Autodesk Fusion 360 part; units mm, degrees
(part 2 of 3)
sketch "Road Junction Left" plane through (0, 0, 0) normal (0, 0, 1) x (1, 0, 0) in component "Road Juntcion left"
  line L0 (106.7005, 11.7668) -> (99.7723, -0.2332)
  line L1 (120.6146, 11.8668) -> (106.6427, 11.8668)
  line L2 (106.7005, -12.2332) -> (120.5569, -12.2332)
  line L3 (104.1544, -16.6432) -> (123.103, -16.6432)
  line L4 (120.0373, -11.3332) -> (126.4458, -0.2332)
  line L5 (99.6568, -0.2332) -> (106.6427, -12.3332)
  line L6 (94.68, -0.2332) -> (104.1544, -16.6432)
  line L7 (100.8115, -0.2332) -> (107.2201, -11.3332)
  line L8 (107.2201, -11.3332) -> (120.0373, -11.3332)
  line L9 (132.5773, -0.2332) -> (123.103, 16.1768)
  line L10 (127.4851, -0.2332) -> (120.5569, 11.7668)
  line L11 (124.021, 5.7668) -> (103.2364, -6.2332) construction
  line L12 (104.1544, 16.1768) -> (94.68, -0.2332)
  line L13 (103.1498, 5.8168) -> (124.1076, -6.2832) construction
  line L14 (106.6427, -12.3332) -> (120.6146, -12.3332)
  line L15 (120.6146, -12.3332) -> (127.6005, -0.2332)
  line L16 (120.5569, 11.7668) -> (106.7005, 11.7668)
  line L17 (127.6005, -0.2332) -> (120.6146, 11.8668)
  line L18 (123.103, -16.6432) -> (132.5773, -0.2332)
  line L19 (123.103, 16.1768) -> (104.1544, 16.1768)
  line L20 (126.4458, -0.2332) -> (120.0373, 10.8668)
  line L21 (120.5569, -12.2332) -> (127.4851, -0.2332)
  line L22 (106.6427, 11.8668) -> (99.6568, -0.2332)
  line L23 (120.0373, 10.8668) -> (107.2201, 10.8668)
  line L24 (113.6287, 11.7668) -> (113.6287, -12.2332) construction
  line L25 (107.2201, 10.8668) -> (100.8115, -0.2332)
  line L26 (99.7723, -0.2332) -> (106.7005, -12.2332)
  line L27 (101.5158, -1.453) -> (120.7416, 9.647)
  line L28 (106.5158, -10.1133) -> (125.7416, 0.9867)
  line L29 (101.7158, -1.7994) -> (120.9416, 9.3006)
  line L30 (106.3158, -9.7669) -> (125.5416, 1.3331)
  line L31 (118.6287, 10.8668) -> (118.6287, -11.3332)
  line L32 (108.6287, 10.8668) -> (108.6287, -11.3332)
  line L33 (118.2287, 10.8668) -> (118.2287, -11.3332)
  line L34 (109.0287, 10.8668) -> (109.0287, -11.3332)
  point P0 (113.6287, -0.2332)
  dimension "d328_3_1" = 0.1
  dimension "d330_3_1" = 32.82
  dimension "d366_1_1" = 10
  dimension "d369_1_1" = 0.4
  dimension "d421" = 10
  dimension "d422" = 0.4
  constraint horizontal L19
  constraint midpoint L24.start L16
  constraint midpoint L24.end L2
  constraint midpoint L11.start L10
  constraint midpoint L11.end L26
  constraint midpoint L13.start L22
  constraint midpoint L13.end L15
  constraint coincident L7 L27.start
  constraint coincident L20 L27.end
  constraint perpendicular L20 L27
  constraint coincident L7 L28.start
  constraint coincident L20 L28.end
  constraint perpendicular L20 L28
  constraint symmetric L11 L27 L28
  constraint coincident L23 L31.start
  constraint coincident L8 L31.end
  constraint perpendicular L8 L31
  constraint coincident L23 L32.start
  constraint coincident L8 L32.end
  constraint perpendicular L8 L32
  constraint symmetric L24 L31 L32
  measures "d330_3_1" distance of L3 L19
  measures "d366_1_1" distance of L27 L28
  measures "d421" distance of L31 L32
extrude "Cap body'" add sketch "Road Junction Left" along normal blind 4.8 separate body contours L0 L2 L10 L16 L21 L26 | L1 L5 L14 L15 L17 L22 | L3 L6 L9 L12 L18 L19 | L4 L8 L20 L28 L31 | L8 L28 L31 L33 | L20 L28 L30 L31 | L8 L28 L33 L34 | L28 L30 L31 L33 | L20 L29 L30 L31 | L8 L28 L32 L34 | L28 L30 L33 L34 | L29 L30 L31 L33 | L20 L27 L29 L31 | L7 L8 L28 L32 | L28 L30 L32 L34 | L29 L30 L33 L34 | L27 L29 L31 L33 | L20 L23 L27 L31 | L7 L28 L30 L32 | L29 L30 L32 L34 | L27 L29 L33 L34 | L23 L27 L31 L33 | L7 L29 L30 L32 | L27 L29 L32 L34 | L23 L27 L33 L34 | L7 L27 L29 L32 | L23 L27 L32 L34 | L7 L23 L25 L27 L32 makes body 9 in component "Road Juntcion left"
extrude "top lip cut''''" cut sketch "Road Junction Left" against normal blind 1.8 from surface at 4.8 contours L1 L5 L14 L15 L17 L22 | L3 L6 L9 L12 L18 L19 bodies 9 in component "Road Juntcion left"
extrude "Cap internal hole'" cut sketch "Road Junction Left" along normal blind 2 contours L0 L2 L10 L16 L21 L26 | L1 L5 L14 L15 L17 L22 | L4 L8 L20 L28 L31 | L8 L28 L31 L33 | L20 L28 L30 L31 | L8 L28 L33 L34 | L28 L30 L31 L33 | L20 L29 L30 L31 | L8 L28 L32 L34 | L28 L30 L33 L34 | L29 L30 L31 L33 | L20 L27 L29 L31 | L7 L8 L28 L32 | L28 L30 L32 L34 | L29 L30 L33 L34 | L27 L29 L31 L33 | L20 L23 L27 L31 | L7 L28 L30 L32 | L29 L30 L32 L34 | L27 L29 L33 L34 | L23 L27 L31 L33 | L7 L29 L30 L32 | L27 L29 L32 L34 | L23 L27 L33 L34 | L7 L27 L29 L32 | L23 L27 L32 L34 | L7 L23 L25 L27 L32 bodies 9 in component "Road Juntcion left"
extrude "road cut'''" cut sketch "Road Junction Left" against normal blind 1.2 from surface at 4.8 contours L4 L8 L20 L28 L31 | L8 L28 L31 L33 | L8 L28 L33 L34 | L8 L28 L32 L34 | L7 L8 L28 L32 | L20 L23 L27 L31 | L7 L23 L25 L27 L32 bodies 9 in component "Road Juntcion left"
extrude "Road depth cut" cut sketch "Road Junction Left" against normal blind 0.4 from surface at 4.8 contours L20 L29 L30 L31 | L29 L30 L31 L33 | L29 L30 L33 L34 | L29 L30 L32 L34 | L27 L29 L33 L34 | L7 L29 L30 L32 | L23 L27 L33 L34 bodies 9 in component "Road Juntcion left"
sketch "Road Junction X" plane through (0, 0, 0) normal (0, 0, 1) x (1, 0, 0) in component "Road Juntcion X"
  line L0 (106.7005, 11.7668) -> (99.7723, -0.2332)
  line L1 (120.6146, 11.8668) -> (106.6427, 11.8668)
  line L2 (106.7005, -12.2332) -> (120.5569, -12.2332)
  line L3 (104.1544, -16.6432) -> (123.103, -16.6432)
  line L4 (120.0373, -11.3332) -> (126.4458, -0.2332)
  line L5 (99.6568, -0.2332) -> (106.6427, -12.3332)
  line L6 (94.68, -0.2332) -> (104.1544, -16.6432)
  line L7 (100.8115, -0.2332) -> (107.2201, -11.3332)
  line L8 (107.2201, -11.3332) -> (120.0373, -11.3332)
  line L9 (132.5773, -0.2332) -> (123.103, 16.1768)
  line L10 (127.4851, -0.2332) -> (120.5569, 11.7668)
  line L11 (124.021, 5.7668) -> (103.2364, -6.2332) construction
  line L12 (104.1544, 16.1768) -> (94.68, -0.2332)
  line L13 (103.1498, 5.8168) -> (124.1076, -6.2832) construction
  line L14 (106.6427, -12.3332) -> (120.6146, -12.3332)
  line L15 (120.6146, -12.3332) -> (127.6005, -0.2332)
  line L16 (120.5569, 11.7668) -> (106.7005, 11.7668)
  line L17 (127.6005, -0.2332) -> (120.6146, 11.8668)
  line L18 (123.103, -16.6432) -> (132.5773, -0.2332)
  line L19 (123.103, 16.1768) -> (104.1544, 16.1768)
  line L20 (126.4458, -0.2332) -> (120.0373, 10.8668)
  line L21 (120.5569, -12.2332) -> (127.4851, -0.2332)
  line L22 (106.6427, 11.8668) -> (99.6568, -0.2332)
  line L23 (120.0373, 10.8668) -> (107.2201, 10.8668)
  line L24 (113.6287, 11.7668) -> (113.6287, -12.2332) construction
  line L25 (107.2201, 10.8668) -> (100.8115, -0.2332)
  line L26 (99.7723, -0.2332) -> (106.7005, -12.2332)
  line L27 (101.5158, -1.453) -> (120.7416, 9.647)
  line L28 (106.5158, -10.1133) -> (125.7416, 0.9867)
  line L29 (101.7158, -1.7994) -> (120.9416, 9.3006)
  line L30 (106.3158, -9.7669) -> (125.5416, 1.3331)
  line L31 (118.6287, 10.8668) -> (118.6287, -11.3332)
  line L32 (108.6287, 10.8668) -> (108.6287, -11.3332)
  line L33 (118.2287, 10.8668) -> (118.2287, -11.3332)
  line L34 (109.0287, 10.8668) -> (109.0287, -11.3332)
  point P0 (113.6287, -0.2332)
  dimension "d328_3_1_1" = 0.1
  dimension "d330_3_1_1" = 32.82
  dimension "d366_1_1_1" = 10
  dimension "d369_1_1_1" = 0.4
  dimension "d421_1" = 10
  dimension "d422_1" = 0.4
  constraint horizontal L19
  constraint midpoint L24.start L16
  constraint midpoint L24.end L2
  constraint midpoint L11.start L10
  constraint midpoint L11.end L26
  constraint midpoint L13.start L22
  constraint midpoint L13.end L15
  constraint coincident L7 L27.start
  constraint coincident L20 L27.end
  constraint perpendicular L20 L27
  constraint coincident L7 L28.start
  constraint coincident L20 L28.end
  constraint perpendicular L20 L28
  constraint symmetric L11 L27 L28
  constraint coincident L23 L31.start
  constraint coincident L8 L31.end
  constraint perpendicular L8 L31
  constraint coincident L23 L32.start
  constraint coincident L8 L32.end
  constraint perpendicular L8 L32
  constraint symmetric L24 L31 L32
  measures "d330_3_1_1" distance of L3 L19
  measures "d366_1_1_1" distance of L27 L28
  measures "d421_1" distance of L31 L32
extrude "Cap body''" add sketch "Road Junction X" along normal blind 4.8 separate body contours L0 L2 L10 L16 L21 L26 | L1 L5 L14 L15 L17 L22 | L3 L6 L9 L12 L18 L19 | L4 L8 L20 L28 L31 | L8 L28 L31 L33 | L20 L28 L30 L31 | L8 L28 L33 L34 | L28 L30 L31 L33 | L20 L29 L30 L31 | L8 L28 L32 L34 | L28 L30 L33 L34 | L29 L30 L31 L33 | L20 L27 L29 L31 | L7 L8 L28 L32 | L28 L30 L32 L34 | L29 L30 L33 L34 | L27 L29 L31 L33 | L20 L23 L27 L31 | L7 L28 L30 L32 | L29 L30 L32 L34 | L27 L29 L33 L34 | L23 L27 L31 L33 | L7 L29 L30 L32 | L27 L29 L32 L34 | L23 L27 L33 L34 | L7 L27 L29 L32 | L23 L27 L32 L34 | L7 L23 L25 L27 L32 makes body 10 in component "Road Juntcion X"
extrude "top lip cut'''''" cut sketch "Road Junction X" against normal blind 1.8 from surface at 4.8 contours L1 L5 L14 L15 L17 L22 | L3 L6 L9 L12 L18 L19 bodies 10 in component "Road Juntcion X"
extrude "Cap internal hole''" cut sketch "Road Junction X" along normal blind 2 contours L0 L2 L10 L16 L21 L26 | L1 L5 L14 L15 L17 L22 | L4 L8 L20 L28 L31 | L8 L28 L31 L33 | L20 L28 L30 L31 | L8 L28 L33 L34 | L28 L30 L31 L33 | L20 L29 L30 L31 | L8 L28 L32 L34 | L28 L30 L33 L34 | L29 L30 L31 L33 | L20 L27 L29 L31 | L7 L8 L28 L32 | L28 L30 L32 L34 | L29 L30 L33 L34 | L27 L29 L31 L33 | L20 L23 L27 L31 | L7 L28 L30 L32 | L29 L30 L32 L34 | L27 L29 L33 L34 | L23 L27 L31 L33 | L7 L29 L30 L32 | L27 L29 L32 L34 | L23 L27 L33 L34 | L7 L27 L29 L32 | L23 L27 L32 L34 | L7 L23 L25 L27 L32 bodies 10 in component "Road Juntcion X"
extrude "road cut''''" cut sketch "Road Junction X" against normal blind 1.2 from surface at 4.8 contours L4 L8 L20 L28 L31 | L7 L8 L28 L32 | L20 L23 L27 L31 | L7 L23 L25 L27 L32 bodies 10 in component "Road Juntcion X"
extrude "Extrude17" cut sketch "Road Junction X" against normal blind 0.4 from surface at 4.8 contours L8 L28 L33 L34 | L20 L29 L30 L31 | L28 L30 L33 L34 | L29 L30 L31 L33 | L29 L30 L33 L34 | L29 L30 L32 L34 | L27 L29 L33 L34 | L7 L29 L30 L32 | L23 L27 L33 L34 bodies 10 in component "Road Juntcion X"
sketch "Road Junction Y" plane through (0, 0, 0) normal (0, 0, 1) x (1, 0, 0) in component "Road Juntcion Y"
  line L0 (106.6902, 11.7491) -> (99.762, -0.2509)
  line L1 (120.6044, 11.8491) -> (106.6325, 11.8491)
  line L2 (106.6902, -12.2509) -> (120.5466, -12.2509)
  line L3 (104.1441, -16.6609) -> (123.0928, -16.6609)
  line L4 (120.027, -11.3509) -> (126.4356, -0.2509)
  line L5 (99.6466, -0.2509) -> (106.6325, -12.3509)
  line L6 (94.6698, -0.2509) -> (104.1441, -16.6609)
  line L7 (100.8013, -0.2509) -> (107.2099, -11.3509)
  line L8 (107.2099, -11.3509) -> (120.027, -11.3509)
  line L9 (132.5671, -0.2509) -> (123.0928, 16.1591)
  line L10 (127.4748, -0.2509) -> (120.5466, 11.7491)
  line L11 (124.0107, 5.7491) -> (103.2261, -6.2509) construction
  line L12 (104.1441, 16.1591) -> (94.6698, -0.2509)
  line L13 (103.1395, 5.7991) -> (124.0973, -6.3009) construction
  line L14 (106.6325, -12.3509) -> (120.6044, -12.3509)
  line L15 (120.6044, -12.3509) -> (127.5903, -0.2509)
  line L16 (120.5466, 11.7491) -> (106.6902, 11.7491)
  line L17 (127.5903, -0.2509) -> (120.6044, 11.8491)
  line L18 (123.0928, -16.6609) -> (132.5671, -0.2509)
  line L19 (123.0928, 16.1591) -> (104.1441, 16.1591)
  line L20 (126.4356, -0.2509) -> (120.027, 10.8491)
  line L21 (120.5466, -12.2509) -> (127.4748, -0.2509)
  line L22 (106.6325, 11.8491) -> (99.6466, -0.2509)
  line L23 (120.027, 10.8491) -> (107.2099, 10.8491)
  line L24 (113.6184, 11.7491) -> (113.6184, -12.2509) construction
  line L25 (107.2099, 10.8491) -> (100.8013, -0.2509)
  line L26 (99.762, -0.2509) -> (106.6902, -12.2509)
  line L27 (101.5056, -1.4708) -> (120.7313, 9.6292)
  line L28 (106.5056, -10.131) -> (125.7313, 0.969)
  line L29 (101.7056, -1.8172) -> (120.9313, 9.2828)
  line L30 (106.3056, -9.7846) -> (125.5313, 1.3154)
  line L31 (118.6184, 10.8491) -> (118.6184, -11.3509)
  line L32 (108.6184, 10.8491) -> (108.6184, -11.3509)
  line L33 (118.2184, 10.8491) -> (118.2184, -11.3509)
  line L34 (109.0184, 10.8491) -> (109.0184, -11.3509)
  line L35 (125.7313, -1.4708) -> (106.5056, 9.6292)
  line L36 (120.7313, -10.131) -> (101.5056, 0.969)
  line L37 (125.5313, -1.8172) -> (106.3056, 9.2828)
  line L38 (120.9313, -9.7846) -> (101.7056, 1.3154)
  point P0 (113.6184, -0.2509)
  dimension "d328_3_1_1_1" = 0.1
  dimension "d330_3_1_1_1" = 32.82
  dimension "d366_1_1_1_1" = 10
  dimension "d369_1_1_1_1" = 0.4
  dimension "d421_1_1" = 10
  dimension "d422_1_1" = 0.4
  dimension "d436" = 10
  dimension "d438" = 0.4
  constraint horizontal L19
  constraint midpoint L24.start L16
  constraint midpoint L24.end L2
  constraint midpoint L11.start L10
  constraint midpoint L11.end L26
  constraint midpoint L13.start L22
  constraint midpoint L13.end L15
  constraint coincident L7 L27.start
  constraint coincident L20 L27.end
  constraint perpendicular L20 L27
  constraint coincident L7 L28.start
  constraint coincident L20 L28.end
  constraint perpendicular L20 L28
  constraint symmetric L11 L27 L28
  constraint coincident L23 L31.start
  constraint coincident L8 L31.end
  constraint perpendicular L8 L31
  constraint coincident L23 L32.start
  constraint coincident L8 L32.end
  constraint perpendicular L8 L32
  constraint symmetric L24 L31 L32
  constraint coincident L4 L35.start
  constraint coincident L25 L35.end
  constraint perpendicular L25 L35
  constraint coincident L4 L36.start
  constraint coincident L25 L36.end
  constraint perpendicular L25 L36
  constraint symmetric L13 L35 L36
  measures "d330_3_1_1_1" distance of L3 L19
  measures "d366_1_1_1_1" distance of L27 L28
  measures "d421_1_1" distance of L31 L32
  measures "d436" distance of L35 L36
extrude "Cap body'''" add sketch "Road Junction Y" along normal blind 4.8 separate body contours L0 L2 L10 L16 L21 L26 | L1 L5 L14 L15 L17 L22 | L3 L6 L9 L12 L18 L19 | L4 L8 L31 L36 | L4 L31 L36 L38 | L8 L31 L33 L36 | L4 L28 L31 L37 L38 | L31 L33 L36 L38 | L8 L28 L33 L34 L36 | L4 L28 L35 L37 | L28 L31 L33 L38 | L28 L33 L36 L38 | L8 L28 L32 L34 | L4 L20 L28 L35 | L28 L30 L35 L37 | L28 L30 L31 L37 | L28 L30 L31 L33 | L28 L33 L38 | L28 L30 L36 L38 | L28 L30 L34 L36 | L7 L8 L28 L32 | L28 L30 L32 L34 | L20 L28 L30 L35 | L30 L31 L35 L37 | L30 L31 L37 | L28 L30 L33 L38 | L30 L31 L33 L37 | L30 L34 L36 L38 | L30 L34 L36 | L7 L28 L30 L32 | L30 L32 L34 L36 | L20 L29 L30 L31 L35 | L31 L33 L35 L37 | L29 L30 L33 L34 L37 L38 | L32 L34 L36 L38 | L7 L29 L30 L32 L36 | L29 L31 L33 L35 | L29 L33 L35 L37 | L29 L32 L34 L38 | L29 L32 L36 L38 | L20 L27 L29 L31 | L27 L29 L31 L33 | L29 L33 L35 | L27 L29 L35 L37 | L27 L29 L34 L37 | L27 L29 L32 L34 | L29 L32 L38 | L27 L29 L36 L38 | L7 L27 L29 L36 | L20 L23 L27 L31 | L27 L29 L33 L35 | L23 L27 L31 L33 | L27 L34 L35 L37 | L27 L34 L37 | L27 L29 L32 L38 | L27 L32 L34 L37 | L25 L27 L36 L38 | L7 L25 L27 L36 | L23 L27 L33 L34 L35 | L32 L34 L35 L37 | L25 L27 L32 L37 L38 | L23 L32 L34 L35 | L25 L32 L35 L37 | L23 L25 L32 L35 makes body 11 in component "Road Juntcion Y"
extrude "top lip cut''''''" cut sketch "Road Junction Y" against normal blind 1.8 from surface at 4.8 contours L1 L5 L14 L15 L17 L22 | L3 L6 L9 L12 L18 L19 bodies 11 in component "Road Juntcion Y"
extrude "Cap internal hole'''" cut sketch "Road Junction Y" along normal blind 2 contours L0 L2 L10 L16 L21 L26 | L1 L5 L14 L15 L17 L22 | L4 L8 L31 L36 | L4 L31 L36 L38 | L8 L31 L33 L36 | L4 L28 L31 L37 L38 | L31 L33 L36 L38 | L8 L28 L33 L34 L36 | L4 L28 L35 L37 | L28 L31 L33 L38 | L28 L33 L36 L38 | L8 L28 L32 L34 | L4 L20 L28 L35 | L28 L30 L35 L37 | L28 L30 L31 L37 | L28 L30 L31 L33 | L28 L33 L38 | L28 L30 L36 L38 | L28 L30 L34 L36 | L7 L8 L28 L32 | L28 L30 L32 L34 | L20 L28 L30 L35 | L30 L31 L35 L37 | L30 L31 L37 | L28 L30 L33 L38 | L30 L31 L33 L37 | L30 L34 L36 L38 | L30 L34 L36 | L7 L28 L30 L32 | L30 L32 L34 L36 | L20 L29 L30 L31 L35 | L31 L33 L35 L37 | L29 L30 L33 L34 L37 L38 | L32 L34 L36 L38 | L7 L29 L30 L32 L36 | L29 L31 L33 L35 | L29 L33 L35 L37 | L29 L32 L34 L38 | L29 L32 L36 L38 | L20 L27 L29 L31 | L27 L29 L31 L33 | L29 L33 L35 | L27 L29 L35 L37 | L27 L29 L34 L37 | L27 L29 L32 L34 | L29 L32 L38 | L27 L29 L36 L38 | L7 L27 L29 L36 | L20 L23 L27 L31 | L27 L29 L33 L35 | L23 L27 L31 L33 | L27 L34 L35 L37 | L27 L34 L37 | L27 L29 L32 L38 | L27 L32 L34 L37 | L25 L27 L36 L38 | L7 L25 L27 L36 | L23 L27 L33 L34 L35 | L32 L34 L35 L37 | L25 L27 L32 L37 L38 | L23 L32 L34 L35 | L25 L32 L35 L37 | L23 L25 L32 L35 bodies 11 in component "Road Juntcion Y"
extrude "road cut'''''" cut sketch "Road Junction Y" against normal blind 1.2 from surface at 4.8 contours L4 L8 L31 L36 | L8 L31 L33 L36 | L8 L28 L33 L34 L36 | L8 L28 L32 L34 | L4 L20 L28 L35 | L7 L8 L28 L32 | L20 L28 L30 L35 | L20 L29 L30 L31 L35 | L20 L27 L29 L31 | L20 L23 L27 L31 | L25 L27 L36 L38 | L7 L25 L27 L36 | L25 L27 L32 L37 L38 | L25 L32 L35 L37 | L23 L25 L32 L35 bodies 11 in component "Road Juntcion Y"
extrude "road depth cut" cut sketch "Road Junction Y" against normal blind 0.4 from surface at 4.8 contours L4 L28 L31 L37 L38 | L28 L31 L33 L38 | L28 L30 L31 L37 | L28 L30 L31 L33 | L28 L33 L38 | L30 L31 L37 | L28 L30 L33 L38 | L30 L31 L33 L37 | L30 L34 L36 L38 | L30 L34 L36 | L30 L32 L34 L36 | L29 L30 L33 L34 L37 L38 | L32 L34 L36 L38 | L7 L29 L30 L32 L36 | L29 L33 L35 L37 | L29 L32 L34 L38 | L29 L32 L36 L38 | L29 L33 L35 | L27 L29 L35 L37 | L27 L29 L34 L37 | L29 L32 L38 | L27 L29 L33 L35 | L27 L34 L35 L37 | L27 L34 L37 | L23 L27 L33 L34 L35 bodies 11 in component "Road Juntcion Y"
sketch "Road Junction Y+I" plane through (0, 0, 0) normal (0, 0, 1) x (1, 0, 0) in component "Road Juntcion Y+I"
  line L0 (106.6902, 11.7491) -> (99.762, -0.2509)
  line L1 (120.6044, 11.8491) -> (106.6325, 11.8491)
  line L2 (106.6902, -12.2509) -> (120.5466, -12.2509)
  line L3 (104.1441, -16.6609) -> (123.0928, -16.6609)
  line L4 (120.027, -11.3509) -> (126.4356, -0.2509)
  line L5 (99.6466, -0.2509) -> (106.6325, -12.3509)
  line L6 (94.6698, -0.2509) -> (104.1441, -16.6609)
  line L7 (100.8013, -0.2509) -> (107.2099, -11.3509)
  line L8 (107.2099, -11.3509) -> (120.027, -11.3509)
  line L9 (132.5671, -0.2509) -> (123.0928, 16.1591)
  line L10 (127.4748, -0.2509) -> (120.5466, 11.7491)
  line L11 (124.0107, 5.7491) -> (103.2261, -6.2509) construction
  line L12 (104.1441, 16.1591) -> (94.6698, -0.2509)
  line L13 (103.1395, 5.7991) -> (124.0973, -6.3009) construction
  line L14 (106.6325, -12.3509) -> (120.6044, -12.3509)
  line L15 (120.6044, -12.3509) -> (127.5903, -0.2509)
  line L16 (120.5466, 11.7491) -> (106.6902, 11.7491)
  line L17 (127.5903, -0.2509) -> (120.6044, 11.8491)
  line L18 (123.0928, -16.6609) -> (132.5671, -0.2509)
  line L19 (123.0928, 16.1591) -> (104.1441, 16.1591)
  line L20 (126.4356, -0.2509) -> (120.027, 10.8491)
  line L21 (120.5466, -12.2509) -> (127.4748, -0.2509)
  line L22 (106.6325, 11.8491) -> (99.6466, -0.2509)
  line L23 (120.027, 10.8491) -> (107.2099, 10.8491)
  line L24 (113.6184, 11.7491) -> (113.6184, -12.2509) construction
  line L25 (107.2099, 10.8491) -> (100.8013, -0.2509)
  line L26 (99.762, -0.2509) -> (106.6902, -12.2509)
  line L27 (101.5056, -1.4708) -> (120.7313, 9.6292)
  line L28 (106.5056, -10.131) -> (125.7313, 0.969)
  line L29 (101.7056, -1.8172) -> (120.9313, 9.2828)
  line L30 (106.3056, -9.7846) -> (125.5313, 1.3154)
  line L31 (118.6184, 10.8491) -> (118.6184, -11.3509)
  line L32 (108.6184, 10.8491) -> (108.6184, -11.3509)
  line L33 (118.2184, 10.8491) -> (118.2184, -11.3509)
  line L34 (109.0184, 10.8491) -> (109.0184, -11.3509)
  line L35 (125.7313, -1.4708) -> (106.5056, 9.6292)
  line L36 (120.7313, -10.131) -> (101.5056, 0.969)
  line L37 (125.5313, -1.8172) -> (106.3056, 9.2828)
  line L38 (120.9313, -9.7846) -> (101.7056, 1.3154)
  point P0 (113.6184, -0.2509)
  dimension "d328_3_1_1_1_1" = 0.1
  dimension "d330_3_1_1_1_1" = 32.82
  dimension "d366_1_1_1_1_1" = 10
  dimension "d369_1_1_1_1_1" = 0.4
  dimension "d421_1_1_1" = 10
  dimension "d422_1_1_1" = 0.4
  dimension "d436_1" = 10
  dimension "d438_1" = 0.4
  constraint horizontal L19
  constraint midpoint L24.start L16
  constraint midpoint L24.end L2
  constraint midpoint L11.start L10
  constraint midpoint L11.end L26
  constraint midpoint L13.start L22
  constraint midpoint L13.end L15
  constraint coincident L7 L27.start
  constraint coincident L20 L27.end
  constraint perpendicular L20 L27
  constraint coincident L7 L28.start
  constraint coincident L20 L28.end
  constraint perpendicular L20 L28
  constraint symmetric L11 L27 L28
  constraint coincident L23 L31.start
  constraint coincident L8 L31.end
  constraint perpendicular L8 L31
  constraint coincident L23 L32.start
  constraint coincident L8 L32.end
  constraint perpendicular L8 L32
  constraint symmetric L24 L31 L32
  constraint coincident L4 L35.start
  constraint coincident L25 L35.end
  constraint perpendicular L25 L35
  constraint coincident L4 L36.start
  constraint coincident L25 L36.end
  constraint perpendicular L25 L36
  constraint symmetric L13 L35 L36
  measures "d330_3_1_1_1_1" distance of L3 L19
  measures "d366_1_1_1_1_1" distance of L27 L28
  measures "d421_1_1_1" distance of L31 L32
  measures "d436_1" distance of L35 L36
extrude "Cap body''''" add sketch "Road Junction Y+I" along normal blind 4.8 separate body contours L0 L2 L10 L16 L21 L26 | L1 L5 L14 L15 L17 L22 | L3 L6 L9 L12 L18 L19 | L4 L8 L31 L36 | L4 L31 L36 L38 | L8 L31 L33 L36 | L4 L28 L31 L37 L38 | L31 L33 L36 L38 | L8 L28 L33 L34 L36 | L4 L28 L35 L37 | L28 L31 L33 L38 | L28 L33 L36 L38 | L8 L28 L32 L34 | L4 L20 L28 L35 | L28 L30 L35 L37 | L28 L30 L31 L37 | L28 L30 L31 L33 | L28 L33 L38 | L28 L30 L36 L38 | L28 L30 L34 L36 | L7 L8 L28 L32 | L28 L30 L32 L34 | L20 L28 L30 L35 | L30 L31 L35 L37 | L30 L31 L37 | L28 L30 L33 L38 | L30 L31 L33 L37 | L30 L34 L36 L38 | L30 L34 L36 | L7 L28 L30 L32 | L30 L32 L34 L36 | L20 L29 L30 L31 L35 | L31 L33 L35 L37 | L29 L30 L33 L34 L37 L38 | L32 L34 L36 L38 | L7 L29 L30 L32 L36 | L29 L31 L33 L35 | L29 L33 L35 L37 | L29 L32 L34 L38 | L29 L32 L36 L38 | L20 L27 L29 L31 | L27 L29 L31 L33 | L29 L33 L35 | L27 L29 L35 L37 | L27 L29 L34 L37 | L27 L29 L32 L34 | L29 L32 L38 | L27 L29 L36 L38 | L7 L27 L29 L36 | L20 L23 L27 L31 | L27 L29 L33 L35 | L23 L27 L31 L33 | L27 L34 L35 L37 | L27 L34 L37 | L27 L29 L32 L38 | L27 L32 L34 L37 | L25 L27 L36 L38 | L7 L25 L27 L36 | L23 L27 L33 L34 L35 | L32 L34 L35 L37 | L25 L27 L32 L37 L38 | L23 L32 L34 L35 | L25 L32 L35 L37 | L23 L25 L32 L35 makes body 12 in component "Road Juntcion Y+I"
extrude "top lip cut'''''''" cut sketch "Road Junction Y+I" against normal blind 1.8 from surface at 4.8 contours L1 L5 L14 L15 L17 L22 | L3 L6 L9 L12 L18 L19 bodies 12 in component "Road Juntcion Y+I"
extrude "Cap internal hole''''" cut sketch "Road Junction Y+I" along normal blind 2 contours L0 L2 L10 L16 L21 L26 | L1 L5 L14 L15 L17 L22 | L4 L8 L31 L36 | L4 L31 L36 L38 | L8 L31 L33 L36 | L4 L28 L31 L37 L38 | L31 L33 L36 L38 | L8 L28 L33 L34 L36 | L4 L28 L35 L37 | L28 L31 L33 L38 | L28 L33 L36 L38 | L8 L28 L32 L34 | L4 L20 L28 L35 | L28 L30 L35 L37 | L28 L30 L31 L37 | L28 L30 L31 L33 | L28 L33 L38 | L28 L30 L36 L38 | L28 L30 L34 L36 | L7 L8 L28 L32 | L28 L30 L32 L34 | L20 L28 L30 L35 | L30 L31 L35 L37 | L30 L31 L37 | L28 L30 L33 L38 | L30 L31 L33 L37 | L30 L34 L36 L38 | L30 L34 L36 | L7 L28 L30 L32 | L30 L32 L34 L36 | L20 L29 L30 L31 L35 | L31 L33 L35 L37 | L29 L30 L33 L34 L37 L38 | L32 L34 L36 L38 | L7 L29 L30 L32 L36 | L29 L31 L33 L35 | L29 L33 L35 L37 | L29 L32 L34 L38 | L29 L32 L36 L38 | L20 L27 L29 L31 | L27 L29 L31 L33 | L29 L33 L35 | L27 L29 L35 L37 | L27 L29 L34 L37 | L27 L29 L32 L34 | L29 L32 L38 | L27 L29 L36 L38 | L7 L27 L29 L36 | L20 L23 L27 L31 | L27 L29 L33 L35 | L23 L27 L31 L33 | L27 L34 L35 L37 | L27 L34 L37 | L27 L29 L32 L38 | L27 L32 L34 L37 | L25 L27 L36 L38 | L7 L25 L27 L36 | L23 L27 L33 L34 L35 | L32 L34 L35 L37 | L25 L27 L32 L37 L38 | L23 L32 L34 L35 | L25 L32 L35 L37 | L23 L25 L32 L35 bodies 12 in component "Road Juntcion Y+I"
extrude "Extrude20" cut sketch "Road Junction Y+I" against normal blind 1.2 from surface at 4.8 contours L4 L8 L31 L36 | L8 L31 L33 L36 | L8 L28 L33 L34 L36 | L8 L28 L32 L34 | L4 L20 L28 L35 | L7 L8 L28 L32 | L20 L23 L27 L31 | L25 L27 L36 L38 | L7 L25 L27 L36 | L25 L27 L32 L37 L38 | L25 L32 L35 L37 | L23 L25 L32 L35 bodies 12 in component "Road Juntcion Y+I"
extrude "Extrude21" cut sketch "Road Junction Y+I" against normal blind 0.4 from surface at 4.8 contours L4 L28 L31 L37 L38 | L28 L31 L33 L38 | L28 L30 L31 L37 | L28 L30 L31 L33 | L28 L33 L38 | L30 L31 L35 L37 | L30 L31 L37 | L28 L30 L33 L38 | L30 L31 L33 L37 | L30 L34 L36 L38 | L30 L34 L36 | L30 L32 L34 L36 | L20 L29 L30 L31 L35 | L31 L33 L35 L37 | L29 L30 L33 L34 L37 L38 | L32 L34 L36 L38 | L7 L29 L30 L32 L36 | L29 L31 L33 L35 | L29 L33 L35 L37 | L29 L32 L34 L38 | L29 L32 L36 L38 | L29 L33 L35 | L27 L29 L35 L37 | L27 L29 L34 L37 | L29 L32 L38 | L27 L29 L33 L35 | L27 L34 L35 L37 | L27 L34 L37 | L23 L27 L33 L34 L35 bodies 12 in component "Road Juntcion Y+I"
sketch "Road Junction X + I" plane through (0, 0, 0) normal (0, 0, 1) x (1, 0, 0) in component "Road Juntcion X + I"
  line L0 (106.6902, 11.7491) -> (99.762, -0.2509)
  line L1 (120.6044, 11.8491) -> (106.6325, 11.8491)
  line L2 (106.6902, -12.2509) -> (120.5466, -12.2509)
  line L3 (104.1441, -16.6609) -> (123.0928, -16.6609)
  line L4 (120.027, -11.3509) -> (126.4356, -0.2509)
  line L5 (99.6466, -0.2509) -> (106.6325, -12.3509)
  line L6 (94.6698, -0.2509) -> (104.1441, -16.6609)
  line L7 (100.8013, -0.2509) -> (107.2099, -11.3509)
  line L8 (107.2099, -11.3509) -> (120.027, -11.3509)
  line L9 (132.5671, -0.2509) -> (123.0928, 16.1591)
  line L10 (127.4748, -0.2509) -> (120.5466, 11.7491)
  line L11 (124.0107, 5.7491) -> (103.2261, -6.2509) construction
  line L12 (104.1441, 16.1591) -> (94.6698, -0.2509)
  line L13 (103.1395, 5.7991) -> (124.0973, -6.3009) construction
  line L14 (106.6325, -12.3509) -> (120.6044, -12.3509)
  line L15 (120.6044, -12.3509) -> (127.5903, -0.2509)
  line L16 (120.5466, 11.7491) -> (106.6902, 11.7491)
  line L17 (127.5903, -0.2509) -> (120.6044, 11.8491)
  line L18 (123.0928, -16.6609) -> (132.5671, -0.2509)
  line L19 (123.0928, 16.1591) -> (104.1441, 16.1591)
  line L20 (126.4356, -0.2509) -> (120.027, 10.8491)
  line L21 (120.5466, -12.2509) -> (127.4748, -0.2509)
  line L22 (106.6325, 11.8491) -> (99.6466, -0.2509)
  line L23 (120.027, 10.8491) -> (107.2099, 10.8491)
  line L24 (113.6184, 11.7491) -> (113.6184, -12.2509) construction
  line L25 (107.2099, 10.8491) -> (100.8013, -0.2509)
  line L26 (99.762, -0.2509) -> (106.6902, -12.2509)
  line L27 (101.5056, -1.4708) -> (120.7313, 9.6292)
  line L28 (106.5056, -10.131) -> (125.7313, 0.969)
  line L29 (101.7056, -1.8172) -> (120.9313, 9.2828)
  line L30 (106.3056, -9.7846) -> (125.5313, 1.3154)
  line L31 (118.6184, 10.8491) -> (118.6184, -11.3509)
  line L32 (108.6184, 10.8491) -> (108.6184, -11.3509)
  line L33 (118.2184, 10.8491) -> (118.2184, -11.3509)
  line L34 (109.0184, 10.8491) -> (109.0184, -11.3509)
  line L35 (125.7313, -1.4708) -> (106.5056, 9.6292)
  line L36 (120.7313, -10.131) -> (101.5056, 0.969)
  line L37 (125.5313, -1.8172) -> (106.3056, 9.2828)
  line L38 (120.9313, -9.7846) -> (101.7056, 1.3154)
  point P0 (113.6184, -0.2509)
  dimension "d328_3_1_1_1_1_1" = 0.1
  dimension "d330_3_1_1_1_1_1" = 32.82
  dimension "d366_1_1_1_1_1_1" = 10
  dimension "d369_1_1_1_1_1_1" = 0.4
  dimension "d421_1_1_1_1" = 10
  dimension "d422_1_1_1_1" = 0.4
  dimension "d436_1_1" = 10
  dimension "d438_1_1" = 0.4
  constraint horizontal L19
  constraint midpoint L24.start L16
  constraint midpoint L24.end L2
  constraint midpoint L11.start L10
  constraint midpoint L11.end L26
  constraint midpoint L13.start L22
  constraint midpoint L13.end L15
  constraint coincident L7 L27.start
  constraint coincident L20 L27.end
  constraint perpendicular L20 L27
  constraint coincident L7 L28.start
  constraint coincident L20 L28.end
  constraint perpendicular L20 L28
  constraint symmetric L11 L27 L28
  constraint coincident L23 L31.start
  constraint coincident L8 L31.end
  constraint perpendicular L8 L31
  constraint coincident L23 L32.start
  constraint coincident L8 L32.end
  constraint perpendicular L8 L32
  constraint symmetric L24 L31 L32
  constraint coincident L4 L35.start
  constraint coincident L25 L35.end
  constraint perpendicular L25 L35
  constraint coincident L4 L36.start
  constraint coincident L25 L36.end
  constraint perpendicular L25 L36
  constraint symmetric L13 L35 L36
  measures "d330_3_1_1_1_1_1" distance of L3 L19
  measures "d366_1_1_1_1_1_1" distance of L27 L28
  measures "d421_1_1_1_1" distance of L31 L32
  measures "d436_1_1" distance of L35 L36
extrude "Cap body'''''" add sketch "Road Junction X + I" along normal blind 4.8 separate body contours L0 L2 L10 L16 L21 L26 | L1 L5 L14 L15 L17 L22 | L3 L6 L9 L12 L18 L19 | L4 L8 L31 L36 | L4 L31 L36 L38 | L8 L31 L33 L36 | L4 L28 L31 L37 L38 | L31 L33 L36 L38 | L8 L28 L33 L34 L36 | L4 L28 L35 L37 | L28 L31 L33 L38 | L28 L33 L36 L38 | L8 L28 L32 L34 | L4 L20 L28 L35 | L28 L30 L35 L37 | L28 L30 L31 L37 | L28 L30 L31 L33 | L28 L33 L38 | L28 L30 L36 L38 | L28 L30 L34 L36 | L7 L8 L28 L32 | L28 L30 L32 L34 | L20 L28 L30 L35 | L30 L31 L35 L37 | L30 L31 L37 | L28 L30 L33 L38 | L30 L31 L33 L37 | L30 L34 L36 L38 | L30 L34 L36 | L7 L28 L30 L32 | L30 L32 L34 L36 | L20 L29 L30 L31 L35 | L31 L33 L35 L37 | L29 L30 L33 L34 L37 L38 | L32 L34 L36 L38 | L7 L29 L30 L32 L36 | L29 L31 L33 L35 | L29 L33 L35 L37 | L29 L32 L34 L38 | L29 L32 L36 L38 | L20 L27 L29 L31 | L27 L29 L31 L33 | L29 L33 L35 | L27 L29 L35 L37 | L27 L29 L34 L37 | L27 L29 L32 L34 | L29 L32 L38 | L27 L29 L36 L38 | L7 L27 L29 L36 | L20 L23 L27 L31 | L27 L29 L33 L35 | L23 L27 L31 L33 | L27 L34 L35 L37 | L27 L34 L37 | L27 L29 L32 L38 | L27 L32 L34 L37 | L25 L27 L36 L38 | L7 L25 L27 L36 | L23 L27 L33 L34 L35 | L32 L34 L35 L37 | L25 L27 L32 L37 L38 | L23 L32 L34 L35 | L25 L32 L35 L37 | L23 L25 L32 L35 makes body 13 in component "Road Juntcion X + I"
extrude "top lip cut''''''''" cut sketch "Road Junction X + I" against normal blind 1.8 from surface at 4.8 contours L1 L5 L14 L15 L17 L22 | L3 L6 L9 L12 L18 L19 bodies 13 in component "Road Juntcion X + I"
extrude "Cap internal hole'''''" cut sketch "Road Junction X + I" along normal blind 2 contours L0 L2 L10 L16 L21 L26 | L1 L5 L14 L15 L17 L22 | L4 L8 L31 L36 | L4 L31 L36 L38 | L8 L31 L33 L36 | L4 L28 L31 L37 L38 | L31 L33 L36 L38 | L8 L28 L33 L34 L36 | L4 L28 L35 L37 | L28 L31 L33 L38 | L28 L33 L36 L38 | L8 L28 L32 L34 | L4 L20 L28 L35 | L28 L30 L35 L37 | L28 L30 L31 L37 | L28 L30 L31 L33 | L28 L33 L38 | L28 L30 L36 L38 | L28 L30 L34 L36 | L7 L8 L28 L32 | L28 L30 L32 L34 | L20 L28 L30 L35 | L30 L31 L35 L37 | L30 L31 L37 | L28 L30 L33 L38 | L30 L31 L33 L37 | L30 L34 L36 L38 | L30 L34 L36 | L7 L28 L30 L32 | L30 L32 L34 L36 | L20 L29 L30 L31 L35 | L31 L33 L35 L37 | L29 L30 L33 L34 L37 L38 | L32 L34 L36 L38 | L7 L29 L30 L32 L36 | L29 L31 L33 L35 | L29 L33 L35 L37 | L29 L32 L34 L38 | L29 L32 L36 L38 | L20 L27 L29 L31 | L27 L29 L31 L33 | L29 L33 L35 | L27 L29 L35 L37 | L27 L29 L34 L37 | L27 L29 L32 L34 | L29 L32 L38 | L27 L29 L36 L38 | L7 L27 L29 L36 | L20 L23 L27 L31 | L27 L29 L33 L35 | L23 L27 L31 L33 | L27 L34 L35 L37 | L27 L34 L37 | L27 L29 L32 L38 | L27 L32 L34 L37 | L25 L27 L36 L38 | L7 L25 L27 L36 | L23 L27 L33 L34 L35 | L32 L34 L35 L37 | L25 L27 L32 L37 L38 | L23 L32 L34 L35 | L25 L32 L35 L37 | L23 L25 L32 L35 bodies 13 in component "Road Juntcion X + I"
extrude "road cut''''''" cut sketch "Road Junction X + I" against normal blind 1.2 from surface at 4.8 contours L4 L8 L31 L36 | L4 L20 L28 L35 | L7 L8 L28 L32 | L20 L23 L27 L31 | L7 L25 L27 L36 | L23 L25 L32 L35 bodies 13 in component "Road Juntcion X + I"
extrude "road indent" cut sketch "Road Junction X + I" against normal blind 0.4 from surface at 4.8 contours L4 L28 L31 L37 L38 | L8 L28 L33 L34 L36 | L28 L31 L33 L38 | L28 L33 L36 L38 | L28 L30 L31 L37 | L28 L30 L31 L33 | L28 L33 L38 | L28 L30 L36 L38 | L28 L30 L34 L36 | L30 L31 L35 L37 | L30 L31 L37 | L28 L30 L33 L38 | L30 L31 L33 L37 | L30 L34 L36 L38 | L30 L34 L36 | L30 L32 L34 L36 | L20 L29 L30 L31 L35 | L31 L33 L35 L37 | L29 L30 L33 L34 L37 L38 | L32 L34 L36 L38 | L7 L29 L30 L32 L36 | L29 L31 L33 L35 | L29 L33 L35 L37 | L29 L32 L34 L38 | L29 L32 L36 L38 | L29 L33 L35 | L27 L29 L35 L37 | L27 L29 L34 L37 | L27 L29 L32 L34 | L29 L32 L38 | L27 L29 L33 L35 | L27 L34 L35 L37 | L27 L34 L37 | L27 L29 L32 L38 | L27 L32 L34 L37 | L23 L27 L33 L34 L35 | L25 L27 L32 L37 L38 bodies 13 in component "Road Juntcion X + I"
sketch "Road Junction 3 Corner" plane through (0, 0, 0) normal (0, 0, 1) x (1, 0, 0) in component "Road Juntcion 3 Corner"
  line L0 (106.6902, 11.7491) -> (99.762, -0.2509)
  line L1 (120.6044, 11.8491) -> (106.6325, 11.8491)
  line L2 (106.6902, -12.2509) -> (120.5466, -12.2509)
  line L3 (104.1441, -16.6609) -> (123.0928, -16.6609)
  line L4 (120.027, -11.3509) -> (126.4356, -0.2509)
  line L5 (99.6466, -0.2509) -> (106.6325, -12.3509)
  line L6 (94.6698, -0.2509) -> (104.1441, -16.6609)
  line L7 (100.8013, -0.2509) -> (107.2099, -11.3509)
  line L8 (107.2099, -11.3509) -> (120.027, -11.3509)
  line L9 (132.5671, -0.2509) -> (123.0928, 16.1591)
  line L10 (127.4748, -0.2509) -> (120.5466, 11.7491)
  line L11 (124.0107, 5.7491) -> (103.2261, -6.2509) construction
  line L12 (104.1441, 16.1591) -> (94.6698, -0.2509)
  line L13 (103.1395, 5.7991) -> (124.0973, -6.3009) construction
  line L14 (106.6325, -12.3509) -> (120.6044, -12.3509)
  line L15 (120.6044, -12.3509) -> (127.5903, -0.2509)
  line L16 (120.5466, 11.7491) -> (106.6902, 11.7491)
  line L17 (127.5903, -0.2509) -> (120.6044, 11.8491)
  line L18 (123.0928, -16.6609) -> (132.5671, -0.2509)
  line L19 (123.0928, 16.1591) -> (104.1441, 16.1591)
  line L20 (126.4356, -0.2509) -> (120.027, 10.8491)
  line L21 (120.5466, -12.2509) -> (127.4748, -0.2509)
  line L22 (106.6325, 11.8491) -> (99.6466, -0.2509)
  line L23 (120.027, 10.8491) -> (107.2099, 10.8491)
  line L24 (113.6184, 11.7491) -> (113.6184, -12.2509) construction
  line L25 (107.2099, 10.8491) -> (100.8013, -0.2509)
  line L26 (99.762, -0.2509) -> (106.6902, -12.2509)
  line L27 (101.5056, -1.4708) -> (120.7313, 9.6292)
  line L28 (106.5056, -10.131) -> (125.7313, 0.969)
  line L29 (101.7056, -1.8172) -> (120.9313, 9.2828)
  line L30 (106.3056, -9.7846) -> (125.5313, 1.3154)
  line L31 (118.6184, 10.8491) -> (118.6184, -11.3509)
  line L32 (108.6184, 10.8491) -> (108.6184, -11.3509)
  line L33 (118.2184, 10.8491) -> (118.2184, -11.3509)
  line L34 (109.0184, 10.8491) -> (109.0184, -11.3509)
  line L35 (125.7313, -1.4708) -> (106.5056, 9.6292)
  line L36 (120.7313, -10.131) -> (101.5056, 0.969)
  line L37 (125.5313, -1.8172) -> (106.3056, 9.2828)
  line L38 (120.9313, -9.7846) -> (101.7056, 1.3154)
  point P0 (113.6184, -0.2509)
  dimension "d328_3_1_1_1_1_1_1" = 0.1
  dimension "d330_3_1_1_1_1_1_1" = 32.82
  dimension "d366_1_1_1_1_1_1_1" = 10
  dimension "d369_1_1_1_1_1_1_1" = 0.4
  dimension "d421_1_1_1_1_1" = 10
  dimension "d422_1_1_1_1_1" = 0.4
  dimension "d436_1_1_1" = 10
  dimension "d438_1_1_1" = 0.4
  constraint horizontal L19
  constraint midpoint L24.start L16
  constraint midpoint L24.end L2
  constraint midpoint L11.start L10
  constraint midpoint L11.end L26
  constraint midpoint L13.start L22
  constraint midpoint L13.end L15
  constraint coincident L7 L27.start
  constraint coincident L20 L27.end
  constraint perpendicular L20 L27
  constraint coincident L7 L28.start
  constraint coincident L20 L28.end
  constraint perpendicular L20 L28
  constraint symmetric L11 L27 L28
  constraint coincident L23 L31.start
  constraint coincident L8 L31.end
  constraint perpendicular L8 L31
  constraint coincident L23 L32.start
  constraint coincident L8 L32.end
  constraint perpendicular L8 L32
  constraint symmetric L24 L31 L32
  constraint coincident L4 L35.start
  constraint coincident L25 L35.end
  constraint perpendicular L25 L35
  constraint coincident L4 L36.start
  constraint coincident L25 L36.end
  constraint perpendicular L25 L36
  constraint symmetric L13 L35 L36
  measures "d330_3_1_1_1_1_1_1" distance of L3 L19
  measures "d366_1_1_1_1_1_1_1" distance of L27 L28
  measures "d421_1_1_1_1_1" distance of L31 L32
  measures "d436_1_1_1" distance of L35 L36
extrude "Cap body''''''" add sketch "Road Junction 3 Corner" along normal blind 4.8 separate body contours L0 L2 L10 L16 L21 L26 | L1 L5 L14 L15 L17 L22 | L3 L6 L9 L12 L18 L19 | L4 L8 L31 L36 | L4 L31 L36 L38 | L8 L31 L33 L36 | L4 L28 L31 L37 L38 | L31 L33 L36 L38 | L8 L28 L33 L34 L36 | L4 L28 L35 L37 | L28 L31 L33 L38 | L28 L33 L36 L38 | L8 L28 L32 L34 | L4 L20 L28 L35 | L28 L30 L35 L37 | L28 L30 L31 L37 | L28 L30 L31 L33 | L28 L33 L38 | L28 L30 L36 L38 | L28 L30 L34 L36 | L7 L8 L28 L32 | L28 L30 L32 L34 | L20 L28 L30 L35 | L30 L31 L35 L37 | L30 L31 L37 | L28 L30 L33 L38 | L30 L31 L33 L37 | L30 L34 L36 L38 | L30 L34 L36 | L7 L28 L30 L32 | L30 L32 L34 L36 | L20 L29 L30 L31 L35 | L31 L33 L35 L37 | L29 L30 L33 L34 L37 L38 | L32 L34 L36 L38 | L7 L29 L30 L32 L36 | L29 L31 L33 L35 | L29 L33 L35 L37 | L29 L32 L34 L38 | L29 L32 L36 L38 | L20 L27 L29 L31 | L27 L29 L31 L33 | L29 L33 L35 | L27 L29 L35 L37 | L27 L29 L34 L37 | L27 L29 L32 L34 | L29 L32 L38 | L27 L29 L36 L38 | L7 L27 L29 L36 | L20 L23 L27 L31 | L27 L29 L33 L35 | L23 L27 L31 L33 | L27 L34 L35 L37 | L27 L34 L37 | L27 L29 L32 L38 | L27 L32 L34 L37 | L25 L27 L36 L38 | L7 L25 L27 L36 | L23 L27 L33 L34 L35 | L32 L34 L35 L37 | L25 L27 L32 L37 L38 | L23 L32 L34 L35 | L25 L32 L35 L37 | L23 L25 L32 L35 makes body 14 in component "Road Juntcion 3 Corner"
extrude "top lip cut'''''''''" cut sketch "Road Junction 3 Corner" against normal blind 1.8 from surface at 4.8 contours L1 L5 L14 L15 L17 L22 | L3 L6 L9 L12 L18 L19 bodies 14 in component "Road Juntcion 3 Corner"
extrude "Cap internal hole''''''" cut sketch "Road Junction 3 Corner" along normal blind 2 contours L0 L2 L10 L16 L21 L26 | L1 L5 L14 L15 L17 L22 | L4 L8 L31 L36 | L4 L31 L36 L38 | L8 L31 L33 L36 | L4 L28 L31 L37 L38 | L31 L33 L36 L38 | L8 L28 L33 L34 L36 | L4 L28 L35 L37 | L28 L31 L33 L38 | L28 L33 L36 L38 | L8 L28 L32 L34 | L4 L20 L28 L35 | L28 L30 L35 L37 | L28 L30 L31 L37 | L28 L30 L31 L33 | L28 L33 L38 | L28 L30 L36 L38 | L28 L30 L34 L36 | L7 L8 L28 L32 | L28 L30 L32 L34 | L20 L28 L30 L35 | L30 L31 L35 L37 | L30 L31 L37 | L28 L30 L33 L38 | L30 L31 L33 L37 | L30 L34 L36 L38 | L30 L34 L36 | L7 L28 L30 L32 | L30 L32 L34 L36 | L20 L29 L30 L31 L35 | L31 L33 L35 L37 | L29 L30 L33 L34 L37 L38 | L32 L34 L36 L38 | L7 L29 L30 L32 L36 | L29 L31 L33 L35 | L29 L33 L35 L37 | L29 L32 L34 L38 | L29 L32 L36 L38 | L20 L27 L29 L31 | L27 L29 L31 L33 | L29 L33 L35 | L27 L29 L35 L37 | L27 L29 L34 L37 | L27 L29 L32 L34 | L29 L32 L38 | L27 L29 L36 L38 | L7 L27 L29 L36 | L20 L23 L27 L31 | L27 L29 L33 L35 | L23 L27 L31 L33 | L27 L34 L35 L37 | L27 L34 L37 | L27 L29 L32 L38 | L27 L32 L34 L37 | L25 L27 L36 L38 | L7 L25 L27 L36 | L23 L27 L33 L34 L35 | L32 L34 L35 L37 | L25 L27 L32 L37 L38 | L23 L32 L34 L35 | L25 L32 L35 L37 | L23 L25 L32 L35 bodies 14 in component "Road Juntcion 3 Corner"
extrude "Extrude24" cut sketch "Road Junction 3 Corner" against normal blind 1.2 from surface at 4.8 contours L4 L8 L31 L36 | L8 L31 L33 L36 | L8 L28 L33 L34 L36 | L8 L28 L32 L34 | L4 L20 L28 L35 | L28 L30 L34 L36 | L7 L8 L28 L32 | L28 L30 L32 L34 | L30 L34 L36 | L7 L28 L30 L32 | L30 L32 L34 L36 | L7 L29 L30 L32 L36 | L29 L32 L36 L38 | L29 L32 L38 | L27 L29 L36 L38 | L7 L27 L29 L36 | L20 L23 L27 L31 | L27 L29 L32 L38 | L25 L27 L36 L38 | L7 L25 L27 L36 | L25 L27 L32 L37 L38 | L25 L32 L35 L37 | L23 L25 L32 L35 bodies 14 in component "Road Juntcion 3 Corner"
extrude "Extrude25" cut sketch "Road Junction 3 Corner" against normal blind 0.4 from surface at 4.8 contours L4 L28 L31 L37 L38 | L28 L31 L33 L38 | L28 L30 L31 L37 | L28 L30 L31 L33 | L28 L33 L38 | L30 L31 L35 L37 | L30 L31 L37 | L28 L30 L33 L38 | L30 L31 L33 L37 | L20 L29 L30 L31 L35 | L31 L33 L35 L37 | L29 L30 L33 L34 L37 L38 | L29 L31 L33 L35 | L29 L33 L35 L37 | L29 L33 L35 | L27 L29 L35 L37 | L27 L29 L34 L37 | L27 L29 L33 L35 | L27 L34 L35 L37 | L27 L34 L37 | L23 L27 L33 L34 L35 bodies 14 in component "Road Juntcion 3 Corner"
sketch "Road Cap Curve Tight" plane through (0, 0, 0) normal (0, 0, 1) x (1, 0, 0) in component "Road Cap Curve tight"
  line L0 (106.898, 12.0938) -> (99.9698, 0.0938)
  line L1 (120.8122, 12.1938) -> (106.8403, 12.1938)
  line L2 (106.898, -11.9062) -> (120.7544, -11.9062)
  line L3 (104.3519, -16.3162) -> (123.3006, -16.3162)
  line L4 (120.2348, -11.0062) -> (126.6434, 0.0938)
  line L5 (99.8544, 0.0938) -> (106.8403, -12.0062)
  line L6 (94.8776, 0.0938) -> (104.3519, -16.3162)
  line L7 (101.0091, 0.0938) -> (107.4176, -11.0062)
  line L8 (107.4176, -11.0062) -> (120.2348, -11.0062)
  line L9 (132.7749, 0.0938) -> (123.3006, 16.5038)
  line L10 (127.6826, 0.0938) -> (120.7544, 12.0938)
  line L11 (124.2185, 6.0938) -> (103.4339, -5.9062) construction
  line L12 (104.3519, 16.5038) -> (94.8776, 0.0938)
  line L13 (103.3473, 6.1438) -> (124.3051, -5.9562) construction
  line L14 (106.8403, -12.0062) -> (120.8122, -12.0062)
  line L15 (120.8122, -12.0062) -> (127.7981, 0.0938)
  line L16 (120.7544, 12.0938) -> (106.898, 12.0938)
  line L17 (127.7981, 0.0938) -> (120.8122, 12.1938)
  line L18 (123.3006, -16.3162) -> (132.7749, 0.0938)
  line L19 (123.3006, 16.5038) -> (104.3519, 16.5038)
  line L20 (126.6434, 0.0938) -> (120.2348, 11.1938)
  line L21 (120.7544, -11.9062) -> (127.6826, 0.0938)
  line L22 (106.8403, 12.1938) -> (99.8544, 0.0938)
  line L23 (120.2348, 11.1938) -> (107.4176, 11.1938)
  line L24 (113.8262, 12.0938) -> (113.8262, -11.9062) construction
  line L25 (107.4176, 11.1938) -> (101.0091, 0.0938)
  line L26 (99.9698, 0.0938) -> (106.898, -11.9062)
  line L27 (123.4391, -5.4562) -> (120.0561, -1.969)
  line L28 (112.4977, -6.3328) -> (113.8262, -11.0062)
  arc A0 (120.0561, -1.969) -> (112.4977, -6.3328) centre (116.8262, -5.1023) ccw
  arc A1 (121.0762, 2.2589) -> (108.3262, -5.1023) centre (116.8262, -5.1023) ccw
  arc A2 (117.1851, -4.7542) -> (116.3453, -5.2391) centre (116.8262, -5.1023) ccw
  line L29 (117.1851, -4.7542) -> (121.3599, -9.0575)
  line L30 (116.3453, -5.2391) -> (117.9847, -11.0062)
  line L31 (121.0762, 2.2589) -> (126.1891, -0.693)
  line L32 (108.3262, -5.1023) -> (108.3262, -11.0062)
  line L33 (120.8762, 1.9125) -> (125.9891, -1.0395)
  line L34 (117.4722, -4.4757) -> (121.647, -8.779)
  line L35 (115.9605, -5.3484) -> (117.6, -11.1156)
  line L36 (108.7262, -5.1023) -> (108.7262, -11.0062)
  arc A3 (120.8762, 1.9125) -> (108.7262, -5.1023) centre (116.8262, -5.1023) ccw
  arc A4 (117.4722, -4.4757) -> (115.9605, -5.3484) centre (116.8262, -5.1023) ccw
  point P0 (113.8262, 0.0938)
  dimension "d328_1_1" = 0.1
  dimension "d330_1_1" = 32.82
  dimension "d463" = 4.5
  dimension "d464" = 5
  dimension "d465" = -5
  dimension "d476" = 0.4
  dimension "d478" = 0.4
  dimension "d481" = 0.4
  constraint horizontal L19
  constraint midpoint L24.start L16
  constraint midpoint L24.end L2
  constraint midpoint L11.start L10
  constraint midpoint L11.end L26
  constraint midpoint L13.start L22
  constraint midpoint L13.end L15
  constraint midpoint L4 L27.start
  constraint midpoint L8 L28.end
  constraint tangent L27 A0
  constraint tangent L28 A0
  constraint coincident L4 L29.end
  constraint tangent A2 L29
  constraint coincident L8 L30.end
  constraint tangent A2 L30
  constraint coincident L4 L31.end
  constraint tangent A1 L31
  constraint coincident L8 L32.end
  constraint tangent A1 L32
  measures "d330_1_1" distance of L3 L19
  measures "d463" radius of A0
extrude "Extrude9''" add sketch "Road Cap Curve Tight" along normal blind 4.8 separate body contours L0 L2 L10 L16 L21 L26 | L1 L5 L14 L15 L17 L22 | L3 L6 L9 L12 L18 L19 | L4 L8 A2 L29 L30 | L4 L8 A2 L29 L30 L34 L35 A4 | L4 L8 L27 L28 A0 L34 L35 A4 | L4 L8 L27 L28 A0 L33 L36 A3 | L4 L8 A1 L31 L32 L33 L36 A3 | L4 L7 L8 L20 L23 L25 A1 L31 L32 makes body 15 in component "Road Cap Curve tight"
extrude "top lip cut''''''''''" cut sketch "Road Cap Curve Tight" against normal blind 1.8 from surface at 4.8 contours L1 L5 L14 L15 L17 L22 | L3 L6 L9 L12 L18 L19 bodies 15 in component "Road Cap Curve tight"
extrude "internal hole" cut sketch "Road Cap Curve Tight" along normal blind 1.8 contours L0 L2 L10 L16 L21 L26 | L1 L5 L14 L15 L17 L22 | L4 L8 A2 L29 L30 | L4 L8 A2 L29 L30 L34 L35 A4 | L4 L8 L27 L28 A0 L34 L35 A4 | L4 L8 L27 L28 A0 L33 L36 A3 | L4 L8 A1 L31 L32 L33 L36 A3 | L4 L7 L8 L20 L23 L25 A1 L31 L32 bodies 15 in component "Road Cap Curve tight"
extrude "Extrude12" cut sketch "Road Cap Curve Tight" against normal blind 1.2 from surface at 4.8 contours L4 L8 A2 L29 L30 | L4 L7 L8 L20 L23 L25 A1 L31 L32 bodies 15 in component "Road Cap Curve tight"
extrude "Extrude13" cut sketch "Road Cap Curve Tight" against normal blind 0.4 from surface at 4.8 contours L4 L8 L27 L28 A0 L34 L35 A4 | L4 L8 L27 L28 A0 L33 L36 A3 bodies 15 in component "Road Cap Curve tight"
component "Basic Cap (Text)" placed x (1, 0, 0) y (0, 1, 0) z (0, 0, 1) at (19.6799, -3.9665, -13.0649)
component "Slab" placed x (1, 0, 0) y (0, 1, 0) z (0, 0, 1) at (0, 0, 0)
component "Multi height Hex" placed x (1, 0, 0) y (0, 1, 0) z (0, 0, 1) at (-60, 0, 0)
component "Basic Hext Tile" placed x (1, 0, 0) y (0, 1, 0) z (0, 0, 1) at (0, 0, 0)
component "Road Cap" placed x (1, 0, 0) y (0, 1, 0) z (0, 0, 1) at (0, 0, 0)
component "Road Cap Curve" placed x (1, 0, 0) y (0, 1, 0) z (0, 0, 1) at (57, 0, 0)
component "Road Cap Bridge" placed x (1, 0, 0) y (0, 1, 0) z (0, 0, 1) at (0, -49, 0)
component "Road Juntcion right" placed x (1, 0, 0) y (0, 1, 0) z (0, 0, 1) at (0, 45, 0)
component "Road Juntcion left" placed x (1, 0, 0) y (0, 1, 0) z (0, 0, 1) at (0, 90, 0)
component "Road Juntcion X" placed x (1, 0, 0) y (0, 1, 0) z (0, 0, 1) at (0, 135, 0)
component "Road Juntcion Y" placed x (1, 0, 0) y (0, 1, 0) z (0, 0, 1) at (0, 179, 0)
component "Road Juntcion Y+I" placed x (1, 0, 0) y (0, 1, 0) z (0, 0, 1) at (0, 222, 0)
component "Road Juntcion X + I" placed x (1, 0, 0) y (0, 1, 0) z (0, 0, 1) at (0, 266, 0)
component "Road Juntcion 3 Corner" placed x (1, 0, 0) y (0, 1, 0) z (0, 0, 1) at (0, 311, 0)
component "Road Cap Curve tight" placed x (1, 0, 0) y (0, 1, 0) z (0, 0, 1) at (130, 0, 0)
equation "hex_size_side_to_side = 32.82 mm"
equation "hex_height = 15 mm"
equation "hex_dt_fem_width_tolerance = 1.2 mm"
equation "d4 = hex_size_side_to_side"
equation "hex_dt_male_width_narrower_part = 5.8 mm"
equation "hex_dt_male_depth = 2.6 mm"
equation "hex_top_lip_width = 4.41 mm"
equation "d16 = -hex_top_lip_width"
equation "hex_wall_thickness = 3.6 mm"
equation "hex_dt_angle = 60 deg"
equation "d29 = hex_dt_male_width_narrower_part"
equation "d31 = hex_dt_male_depth"
equation "d32 = hex_dt_angle"
equation "d34 = hex_dt_male_width_narrower_part + hex_dt_fem_width_tolerance"
equation "d35 = hex_dt_angle"
equation "d38 = hex_height"
equation "d41 = -hex_top_lip_height"
equation "d44 = hex_dt_male_depth + hex_dt_fem_depth_tolerance"
equation "hex_top_lip_height = 2 mm"
equation "hex_dt_fem_depth_tolerance = 0.4 mm"
equation "hex_dt_male_bottom_distance = 5 mm"
equation "d51 = hex_dt_male_bottom_distance + hex_dt_spacing_height_tolerance"
equation "hex_dt_spacing_height_tolerance = 1 mm"
equation "hex_internal_hole_height = 11 mm"
equation "hex_internal_hole_offset = 0.1 mm" comment "Diferencia entre el agujero y el hex de la parte superior"
equation "d59 = hex_internal_hole_offset"
equation "d60 = hex_internal_hole_height"
equation "d62 = hex_internal_hole_height"
equation "cap_height = ( hex_top_lip_height * 2 ) + cap_height_tolerance"
equation "cap_height_tolerance = 0.8 mm"
equation "d65_1 = hex_size_side_to_side"
equation "d66_1 = -hex_top_lip_width"
equation "d67_1 = hex_internal_hole_offset"
equation "d88 = cap_text_height"
equation "d89 = cap_text"
equation "cap_text = '+3\\nWATER3\\nPSR+1'"
equation "cap_sculpted_top_wall_thickness = 1 mm"
equation "cap_sculpted_hole_depth = 1.2 mm"
equation "d100 = -cap_sculpted_top_wall_thickness"
equation "cap_text_height = 4 mm"
equation "slab_v_spacing = hex_size_side_to_side * 0.866025"
equation "slab_h_offset = hex_size_side_to_side / 2"
equation "slab_h_spacing = hex_size_side_to_side"
equation "slab_base_height = 2 mm"
equation "d210 = cap_height"
equation "d213 = -cap_top_lip_height"
equation "d216 = -cap_sculpted_hole_depth"
equation "d218 = hex_top_lip_height"
equation "d224 = cap_sculpted_hole_depth"
equation "d250 = -hex_top_lip_width"
equation "d256 = -hex_top_lip_width"
equation "d257 = slab_h_offset"
equation "d258 = slab_v_spacing"
equation "d268 = hex_dt_male_depth"
equation "d269 = hex_dt_angle"
equation "d270 = hex_dt_male_width_narrower_part"
equation "d274 = hex_dt_angle"
equation "d275 = hex_dt_male_width_narrower_part"
equation "d276 = hex_dt_male_depth"
equation "d277 = hex_dt_angle"
equation "d278 = hex_dt_male_depth"
equation "d279 = hex_dt_male_width_narrower_part"
equation "d280 = hex_dt_angle"
equation "d281 = hex_dt_male_width_narrower_part"
equation "d282 = hex_dt_male_depth"
equation "d295 = hex_dt_male_width_narrower_part + hex_dt_fem_width_tolerance"
equation "d296 = hex_dt_male_depth + slab_dt_fem_depth_tolerance"
equation "d297 = hex_dt_angle"
equation "d298 = hex_dt_male_width_narrower_part + hex_dt_fem_width_tolerance"
equation "d299 = hex_dt_male_depth + slab_dt_fem_depth_tolerance"
equation "d300 = hex_dt_angle"
equation "d301 = hex_dt_male_width_narrower_part + hex_dt_fem_width_tolerance"